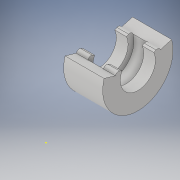
# Autodesk Inventor part: GarraBearing
Saved by Autodesk Inventor 2019 (Build 230136000, 136)
## iProperties
Created: 2020-01-20
Part Number: GarraBearing
Material: Generic
Document SubType Name: Modeling
Designer: peter
Density: 1 g/cm^3
Appearance: Default
Author: peter
Autodesk Inventor part; units mm, degrees
ref_plane "YZ Plane" through (0, 0, 0) normal (1, 0, 0) x (0, 1, 0)
ref_plane "XZ Plane" through (0, 0, 0) normal (0, 1, 0) x (-1, 0, 0)
ref_plane "XY Plane" through (0, 0, 0) normal (0, 0, 1) x (1, 0, 0)
sketch "Sketch2" plane through (0, 0, 0) normal (1, 0, 0) x (0, 1, 0)
  arc A0 (5.9909, -17.7467) -> (5.9909, -29.2731) centre (4.322, -23.5099) ccw
  arc A1 (6.2238, -19.4315) -> (6.2238, -27.5883) centre (4.322, -23.5099) ccw
  line L0 (6.2238, -19.4315) -> (6.4935, -18.8532)
  line L1 (6.2238, -27.5883) -> (6.4935, -28.1666)
  arc A2 (6.4935, -18.8532) -> (5.9909, -17.7467) centre (5.7684, -18.5151) ccw
  arc A3 (5.9909, -29.2731) -> (6.4935, -28.1666) centre (5.7684, -28.5047) ccw
  point P0 (0, 0)
  point P1 (6.8577, -28.9477)
  point P2 (6.8577, -18.072)
  dimension "d1" = 130
  dimension "d2" = 6
  dimension "d5" = 1.5
  dimension "d6" = 0.8
  constraints: 10 point on circle, 4 centre point, 4 end point, 4 tangent, 2 point on line, 1 equal radius
  measures "d2" radius of A0
  measures "d5" radial gap between concentric circles of A0 A1
  measures "d6" radius of A2
extrude "Extrusion1" add sketch "Sketch2" along normal blind 4
shell "Shell1" thickness 3 outward yes removed faces 5 at (2.6667, 1.83, -27.2568) at (1.3333, 6.4036, -19.046) at (2.6667, 6.2793, -17.8995) at (1.3333, 6.3137, -27.781) at (2.6667, 6.3731, -29.0285)
sketch "Sketch5" plane through (7, 0, 0) normal (1, 0, 0) x (0, 0, -1)
  point P0 (0, 0)
sketch "Sketch6" plane through (7, 0, 0) normal (1, 0, 0) x (0, 0, -1)
  point P0 (0, 0)
body "Solid1"
